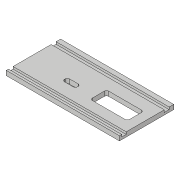
# Autodesk Inventor part: Electronics Container Part 2
Saved by Autodesk Inventor 2018.3 (Build 223284000, 284)
## iProperties
Created: 2019-03-04
Part Number: Electronics Container Part 2
Material: Generic
Document SubType Name: Modeling
Designer: aye06091
Mass: 7.73212 g
Surface Area: 69.2703 cm^2
Volume: 7.73212 cm^3
Density: 1 g/cm^3
Appearance: Default
Author: aye06091
Autodesk Inventor part; units mm, degrees
ref_plane "YZ Plane" through (0, 0, 0) normal (1, 0, 0) x (0, 1, 0)
ref_plane "XZ Plane" through (0, 0, 0) normal (0, 1, 0) x (-1, 0, 0)
ref_plane "XY Plane" through (0, 0, 0) normal (0, 0, 1) x (1, 0, 0)
sketch "Sketch1" plane through (0, 0, 0) normal (0, 1, 0) x (-1, 0, 0)
  line L0 (0, 0) -> (-79.375, 0)
  line L1 (-79.375, 0) -> (-79.375, 38.1)
  line L2 (-79.375, 38.1) -> (0, 38.1)
  line L3 (0, 38.1) -> (0, 0)
  dimension "d0" = 79.375
  dimension "d1" = 38.1
  constraints: 8 end point, 2 parallel, 1 horizontal, 1 perpendicular
  measures "d0" distance of L0.start L0.end
  measures "d1" distance of L2.end L0.start
extrude "Extrusion1" add sketch "Sketch1" along normal blind 3.175
sketch "Sketch2" plane through (0, 3.175, 0) normal (0, 1, 0) x (1, 0, 0)
  line L0 (0, 0) -> (0, -38.1) projected
  line L1 (79.375, -38.1) -> (79.375, 0) projected
  line L2 (0, -33.3121) -> (79.375, -33.3121)
  line L3 (79.375, -33.3121) -> (79.375, -36.5125)
  line L4 (79.375, -36.5125) -> (0, -36.5125)
  line L5 (0, -36.5125) -> (0, -33.3121)
  line L6 (0, -38.1) -> (79.375, -38.1) projected
  line L7 (79.375, 0) -> (0, 0) projected
  line L8 (79.375, -3.175) -> (0, -3.175)
  line L9 (0, -3.175) -> (0, -6.604)
  line L10 (0, -6.604) -> (79.375, -6.604)
  line L11 (79.375, -6.604) -> (79.375, -3.175)
  dimension "d4" = 3.2004
  dimension "d8" = 1.5875
  dimension "d13" = 3.175
  dimension "d14" = 3.429
  constraints: 16 end point, 4 parallel, 4 point on line, 2 horizontal, 2 perpendicular
  measures "d4" distance between parallel lines of L4 L2
  measures "d8" distance between parallel lines of L6 L4
  measures "d13" distance between parallel lines of L7 L8
  measures "d14" distance between parallel lines of L10 L8
extrude "Extrusion2" cut sketch "Sketch2" against normal blind 1.5875 contours L8 L1 L10 L0 | L2 L1 L4 L0
sketch "Sketch4" plane through (0, 3.175, 0) normal (0, 1, 0) x (1, 0, 0)
  line L0 (0, -33.3121) -> (79.375, -33.3121) projected
  line L1 (79.375, -33.3121) -> (79.375, -6.604) projected
  line L2 (25.781, -21.0566) -> (34.925, -21.0566)
  line L3 (34.925, -21.0566) -> (34.925, -24.6126)
  line L4 (34.925, -24.6126) -> (25.781, -24.6126)
  line L5 (25.781, -24.6126) -> (25.781, -21.0566)
  line L6 (46.99, -14.7701) -> (73.025, -14.7701)
  line L7 (73.025, -14.7701) -> (73.025, -26.2001)
  line L8 (73.025, -26.2001) -> (46.99, -26.2001)
  line L9 (46.99, -26.2001) -> (46.99, -14.7701)
  point P0 (0, 0)
  dimension "d15" = 3.556
  dimension "d16" = 9.144
  dimension "d17" = 8.6995
  dimension "d18" = 44.45
  dimension "d19" = 26.035
  dimension "d20" = 11.43
  dimension "d21" = 7.112
  dimension "d22" = 6.35
  constraints: 16 end point, 4 parallel, 2 horizontal, 2 perpendicular
  measures "d15" distance between parallel lines of L2 L4
  measures "d16" distance of L2.start L2.end
  measures "d17" distance between parallel lines of L0 L4
  measures "d18" distance between parallel lines of L1 L3
  measures "d19" distance of L6.start L6.end
  measures "d20" distance of L8.end L6.start
  measures "d21" distance between parallel lines of L0 L8
  measures "d22" distance between parallel lines of L1 L7
extrude "Extrusion4" cut sketch "Sketch4" against normal blind 25.4
fillet "Fillet1" radius 1.5875 4 edges at (25.781, 1.5875, 21.0566) (25.781, 1.5875, 24.6126) (34.925, 1.5875, 24.6126) (34.925, 1.5875, 21.0566)
fillet "Fillet2" radius 1.5875 4 edges at (73.025, 1.5875, 14.7701) (73.025, 1.5875, 26.2001) (46.99, 1.5875, 26.2001) (46.99, 1.5875, 14.7701)
body "Solid1"
